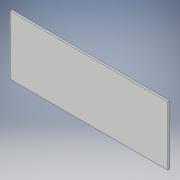
# Autodesk Inventor part: solarpanel
Saved by Autodesk Inventor 2018 (Build 220112000, 112)
## iProperties
Created: 2018-04-24
Part Number: solarpanel
Material: Generic
Document SubType Name: Modeling
Designer: atbin
Mass: 556699 g
Surface Area: 502000 cm^2
Volume: 2.4e+06 cm^3
Density: 0.231958 g/cm^3
Appearance: Default
Author: atbin
Autodesk Inventor part; units mm, degrees
ref_plane "YZ Plane" through (0, 0, 0) normal (1, 0, 0) x (0, 1, 0)
ref_plane "XZ Plane" through (0, 0, 0) normal (0, 1, 0) x (-1, 0, 0)
ref_plane "XY Plane" through (0, 0, 0) normal (0, 0, 1) x (1, 0, 0)
sketch "Sketch1" plane through (0, 0, 0) normal (0, 0, 1) x (1, 0, 0)
  line L0 (-4000, -1500) -> (4000, -1500)
  line L1 (4000, -1500) -> (4000, 1500)
  line L2 (4000, 1500) -> (-4000, 1500)
  line L3 (-4000, 1500) -> (-4000, -1500)
  line L4 (-4000, -1500) -> (4000, 1500) construction
  line L5 (4000, -1500) -> (-4000, 1500) construction
  point P0 (0, 0)
  dimension "d0" = 8000
  dimension "d1" = 3000
  constraints: 12 end point, 2 midpoint, 2 parallel, 1 horizontal, 1 perpendicular
  measures "d0" distance of L1.end L2.end
  measures "d1" distance of L2.end L0.start
extrude "Extrusion1" add sketch "Sketch1" along normal blind 100
body "Solid1"
